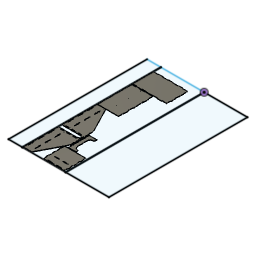
remorque marelle v9.1 v3 (Autodesk Fusion 360 design; units mm, degrees)
Autodesk Fusion 360 part; units mm, degrees
(part 1 of 2)
sketch "Esquisse1" plane through (0, 0, 0) normal (1, 0, 0) x (0, 0, -1)
  line L0 (0, 0) -> (0, 988)
  line L1 (0, 988) -> (-12, 988)
  line L2 (-12, 988) -> (-12, 0)
  line L3 (-12, 0) -> (0, 0)
  line L4 (605, 0) -> (0, 0)
  line L5 (180, 988) -> (192, 988)
  line L6 (192, 988) -> (192, 0)
  line L7 (192, 0) -> (180, 0)
  line L8 (180, 0) -> (180, 988)
  line L9 (-12, 988) -> (192, 988)
  line L10 (-12, 0) -> (605, 0)
  line L11 (605, 0) -> (605, -12)
  line L12 (605, -12) -> (-12, -12)
  line L13 (-12, -12) -> (-12, 0)
  line L14 (192, 988) -> (209.8465, 988)
  line L15 (227.5983, 977.2127) -> (569.8721, 317.6877)
  line L16 (605, 173.7399) -> (605, 0)
  arc A0 (227.5983, 977.2127) -> (209.8465, 988) centre (209.8465, 968) ccw
  arc A1 (605, 173.7399) -> (569.8721, 317.6877) centre (292.5, 173.7399) ccw
  line L17 (0, 988) -> (-12, 988)
  line L18 (-12, 988) -> (-12, 845.1428)
  line L19 (-12, 845.1428) -> (0, 845.1428)
  line L20 (0, 845.1428) -> (0, 988)
  line L21 (-12, 988) -> (-32.1287, 988)
  line L22 (-32.1287, 988) -> (-32.1287, -12)
  line L23 (-32.1287, -12) -> (-12, -12)
  line L24 (-12, -12) -> (-12, 988)
  line L25 (605, -12) -> (-32, -12)
  line L26 (-32, -12) -> (-32, -32)
  line L27 (-32, -32) -> (605, -32)
  line L28 (605, -32) -> (605, -12)
  line L29 (-32, -32) -> (-12, -32)
  line L30 (-12, -32) -> (-12, -12)
  line L31 (-12, -12) -> (-32, -12)
  line L32 (-32, -12) -> (-32, -32)
  line L33 (605, -32) -> (585, -32)
  line L34 (585, -32) -> (585, -12)
  line L35 (585, -12) -> (605, -12)
  line L36 (605, -12) -> (605, -32)
  line L37 (296.5, -12) -> (276.5, -12)
  line L38 (276.5, -12) -> (276.5, -32)
  line L39 (276.5, -32) -> (296.5, -32)
  line L40 (296.5, -32) -> (296.5, -12)
  line L41 (-12, 702.2857) -> (0, 702.2857)
  line L42 (0, 702.2857) -> (0, 845.1428)
  line L43 (-12, 845.1428) -> (-12, 702.2857)
  line L44 (0, 845.1428) -> (-12, 845.1428)
  line L45 (-12, 559.4286) -> (0, 559.4286)
  line L46 (0, 559.4286) -> (0, 702.2857)
  line L47 (-12, 702.2857) -> (-12, 559.4286)
  line L48 (0, 702.2857) -> (-12, 702.2857)
  line L49 (-12, 416.5714) -> (0, 416.5714)
  line L50 (0, 416.5714) -> (0, 559.4286)
  line L51 (-12, 559.4286) -> (-12, 416.5714)
  line L52 (0, 559.4286) -> (-12, 559.4286)
  line L53 (-12, 273.7143) -> (0, 273.7143)
  line L54 (0, 273.7143) -> (0, 416.5714)
  line L55 (-12, 416.5714) -> (-12, 273.7143)
  line L56 (0, 416.5714) -> (-12, 416.5714)
  line L57 (-12, 130.8571) -> (0, 130.8571)
  line L58 (0, 130.8571) -> (0, 273.7143)
  line L59 (-12, 273.7143) -> (-12, 130.8571)
  line L60 (0, 273.7143) -> (-12, 273.7143)
  line L61 (90, 988) -> (90, 0) construction
  line L62 (192, 130.8571) -> (180, 130.8571)
  line L63 (180, 273.7143) -> (192, 273.7143)
  line L64 (180, 416.5714) -> (192, 416.5714)
  line L65 (192, 559.4286) -> (180, 559.4286)
  line L66 (180, 702.2857) -> (192, 702.2857)
  line L67 (180, 845.1428) -> (192, 845.1428)
  line L68 (192, 0) -> (180, 0)
  line L69 (180, 0) -> (180, -12)
  line L70 (180, -12) -> (192, -12)
  line L71 (192, -12) -> (192, 0)
  line L72 (0, 0) -> (0, -12)
  line L73 (605, 0) -> (514, 0)
  line L74 (514, 0) -> (514, -12)
  line L75 (514, -12) -> (605, -12)
  line L76 (605, -12) -> (605, 0)
  line L77 (423, 0) -> (423, -12)
  line L78 (514, -12) -> (514, 0)
  line L79 (332, 0) -> (332, -12)
  line L80 (423, -12) -> (423, 0)
  line L81 (241, 0) -> (241, -12)
  line L82 (332, -12) -> (332, 0)
  line L83 (150, 0) -> (150, -12)
  line L84 (241, -12) -> (241, 0)
  line L85 (59, 0) -> (59, -12)
  line L86 (150, -12) -> (150, 0)
  line L87 (-32, 0) -> (-32, -12)
  line L88 (59, -12) -> (59, 0)
  line L89 (605, 173.7399) -> (593, 173.7399)
  line L90 (593, 173.7399) -> (593, -12)
  line L91 (593, -12) -> (605, -12)
  line L92 (605, -12) -> (605, 173.7399)
  line L93 (593, 173.7399) -> (605, 173.7399)
  line L94 (605, 173.7399) -> (605, 158.7399)
  line L95 (605, 158.7399) -> (593, 158.7399)
  line L96 (593, 158.7399) -> (593, 173.7399)
  line L97 (-12, 0) -> (-32, 0)
  circle A2 centre (-6, 973) radius 2
  circle A3 centre (-6, 860.1428) radius 2
  circle A4 centre (-6, 717.2857) radius 2
  circle A5 centre (-6, 830.1428) radius 2
  circle A6 centre (-6, 574.4286) radius 2
  circle A7 centre (-6, 687.2857) radius 2
  circle A8 centre (-6, 431.5714) radius 2
  circle A9 centre (-6, 544.4286) radius 2
  circle A10 centre (-6, 288.7143) radius 2
  circle A11 centre (-6, 401.5714) radius 2
  circle A12 centre (-6, 145.8571) radius 2
  circle A13 centre (-6, 258.7143) radius 2
  line L98 (-12, -12) -> (0, -12)
  line L99 (0, -12) -> (0, 130.8571)
  line L100 (-12, 130.8571) -> (-12, -12)
  line L101 (0, 130.8571) -> (-12, 130.8571)
  circle A14 centre (-6, 115.8571) radius 2
  circle A15 centre (186, 973) radius 2
  circle A16 centre (186, 860.1428) radius 2
  circle A17 centre (186, 687.2857) radius 2
  circle A18 centre (186, 574.4286) radius 2
  circle A19 centre (186, 401.5714) radius 2
  circle A20 centre (186, 288.7143) radius 2
  circle A21 centre (186, 115.8571) radius 2
  circle A22 centre (186, 15) radius 2
  circle A23 centre (-6, 15) radius 2
  line L102 (605, -6) -> (-32, -6) construction
  circle A24 centre (-20.1287, -6) radius 2
  circle A25 centre (47, -6) radius 2
  circle A26 centre (70.8713, -6) radius 2
  circle A27 centre (138, -6) radius 2
  circle A28 centre (161.8713, -6) radius 2
  circle A29 centre (229, -6) radius 2
  circle A30 centre (252.8713, -6) radius 2
  circle A31 centre (320, -6) radius 2
  circle A32 centre (343.8713, -6) radius 2
  circle A33 centre (411, -6) radius 2
  circle A34 centre (434.8713, -6) radius 2
  circle A35 centre (502, -6) radius 2
  circle A36 centre (525.8713, -6) radius 2
  circle A37 centre (593, -6) radius 2
  circle A38 centre (581, -6) radius 2
  line L103 (599, 158.7399) -> (593, 158.7399)
  line L104 (593, 158.7399) -> (593, 150.7399)
  line L105 (593, 150.7399) -> (599, 150.7399)
  line L106 (599, 150.7399) -> (599, 158.7399)
  point P0 (222, 988)
  point P1 (605, 250)
  dimension "d1" = 12
  dimension "d5" = 12
  dimension "d6" = 180
  dimension "d7" = 413
  dimension "d8" = 12
  dimension "d9" = 250
  dimension "d10" = 30
  dimension "d11" = 20
  dimension "d12" = 312.5
  dimension "d15" = 142.8571
  dimension "d17" = 20
  dimension "d18" = 20
  dimension "d19" = 20
  dimension "d22" = 0
  dimension "d23" = -142.8571
  dimension "d24" = 20
  dimension "d25" = 1020
  dimension "d28" = 91
  dimension "d31" = -91
  dimension "d32" = 0
  dimension "d44" = 12
  dimension "d47" = 15
  dimension "d56" = 4
  dimension "d57" = 6
  dimension "d58" = 15
  dimension "d59" = 4
  dimension "d60" = 15
  dimension "d61" = 6
  dimension "d62" = 4
  dimension "d63" = 15
  dimension "d64" = 4
  dimension "d65" = 15
  dimension "d66" = 4
  dimension "d67" = 4
  dimension "d68" = 12
  dimension "d69" = 12
  dimension "d72" = 91
  dimension "d73" = 0
  dimension "d74" = 4
  dimension "d75" = 12
  dimension "d103" = 8
  constraint coincident L0.start L3.end
  constraint vertical L0
  constraint perpendicular L0 L1
  constraint perpendicular L1 L2
  constraint perpendicular L0 L3
  constraint perpendicular L0 L4
  constraint horizontal L5
  constraint vertical L6
  constraint horizontal L7
  constraint vertical L8
  constraint coincident L4 L6.end
  constraint perpendicular L6 L9
  constraint horizontal L10
  constraint vertical L11
  constraint horizontal L12
  constraint vertical L13
  constraint perpendicular L6 L14
  constraint perpendicular L10 L16
  constraint coincident P0 L14
  constraint coincident P0 L15
  constraint tangent L14 A0
  constraint tangent L15 A0
  constraint coincident P1 L15
  constraint coincident P1 L16
  constraint tangent L15 A1
  constraint tangent L16 A1
  constraint horizontal L17
  constraint vertical L18
  constraint horizontal L19
  constraint vertical L20
  constraint coincident L2 L18.end
  constraint horizontal L21
  constraint vertical L22
  constraint horizontal L23
  constraint vertical L24
  constraint horizontal L25
  constraint vertical L26
  constraint horizontal L27
  constraint vertical L28
  constraint horizontal L29
  constraint vertical L30
  constraint horizontal L31
  constraint vertical L32
  constraint horizontal L33
  constraint vertical L34
  constraint horizontal L35
  constraint vertical L36
  constraint horizontal L37
  constraint vertical L38
  constraint horizontal L39
  constraint vertical L40
  constraint coincident L12 L37.start
  constraint midpoint L27 L39
  constraint midpoint L9 L61.start
  constraint coincident L10 L61.end
  constraint perpendicular L4 L61
  constraint symmetric L19.end L61 L67.start
  constraint symmetric L18.end L61 L67.end
  constraint symmetric L45.start L61 L65.start
  constraint symmetric L45.end L61 L65.end
  constraint symmetric L41.end L61 L66.start
  constraint symmetric L41.start L61 L66.end
  constraint symmetric L49.end L61 L64.start
  constraint symmetric L49.start L61 L64.end
  constraint symmetric L57.start L61 L62.start
  constraint symmetric L57.end L61 L62.end
  constraint symmetric L53.end L61 L63.start
  constraint symmetric L53.start L61 L63.end
  constraint horizontal L68
  constraint vertical L69
  constraint horizontal L70
  constraint vertical L71
  constraint coincident L25 L69.end
  constraint coincident L7.end L8.start
  constraint coincident L12 L72.end
  constraint collinear L0 L72
  constraint horizontal L73
  constraint vertical L74
  constraint horizontal L75
  constraint vertical L76
  constraint coincident L25 L74.end
  constraint coincident L4.start L10.end
  constraint horizontal L89
  constraint vertical L90
  constraint horizontal L91
  constraint vertical L92
  constraint coincident L25 L90.end
  constraint coincident L35 L90.end
  constraint horizontal L93
  constraint vertical L94
  constraint horizontal L95
  constraint vertical L96
  constraint symmetric L61 A2 A15
  constraint symmetric L61 A3 A16
  constraint symmetric L61 A6 A18
  constraint symmetric L61 A7 A17
  constraint symmetric L61 A10 A20
  constraint symmetric L61 A11 A19
  constraint symmetric L61 A14 A21
  constraint midpoint L11 L102.start
  constraint midpoint L87 L102.end
  constraint coincident L102 A24.centre
  constraint coincident L102 A25.centre
  constraint coincident L102 A38.centre
  constraint horizontal L103
  constraint vertical L104
  constraint horizontal L105
  constraint vertical L106
  constraint coincident L90 L104.end
  constraint midpoint L95 L103.start
  measures "d1" distance of L2.end L0.start
  measures "d5" distance of L6 L8
  measures "d6" distance of L0 L8
  measures "d7" distance of L4.start L6
  measures "d8" distance of L10 L12
  measures "d9" distance of L4.start P1
  measures "d10" distance of L5.end P0
  measures "d11" radius of A0
  measures "d12" radius of A1
  measures "d15" distance of L0.end L19.end
  measures "d17" distance of L25 L27
  measures "d18" distance of L27.end L33.end
  measures "d19" distance of L38 L40
  measures "d24" distance of L26 L30
  measures "d25" distance of L21.end L26.end
  measures "d28" distance of L74 L76
  measures "d44" distance of L16 L90
  measures "d47" distance of L89.end L95.end
  measures "d56" diameter of A2
  measures "d57" distance of L18 A2.centre
  measures "d58" distance of L9 A2.centre
  measures "d59" diameter of A3
  measures "d60" distance of L44 A3.centre
  measures "d61" distance of L18 A3.centre
  measures "d62" diameter of A22
  measures "d63" distance of L68 A22.centre
  measures "d64" diameter of A23
  measures "d65" distance of L3 A23.centre
  measures "d66" diameter of A24
  measures "d67" diameter of A25
  measures "d68" distance of L85 A25.centre
  measures "d69" distance of L22 A24.centre
  measures "d74" diameter of A38
  measures "d75" distance of A37.centre A38.centre
  measures "d103" distance of L103.start L105.end
sketch "Esquisse2" plane through (0, 0, 0) normal (1, 0, 0) x (0, 0, -1)
  line L0 (605, -12) -> (-32, -12)
  line L1 (-32, -32) -> (605, -32)
  line L2 (-12, 0) -> (605, 0)
  line L3 (-32, 0) -> (-32, -12)
  line L4 (-32, -12) -> (-32, -32)
  line L5 (605, -12) -> (605, -32)
  line L6 (605, 0) -> (605, -12)
  line L7 (-12, -32) -> (113, -32)
  line L8 (113, -32) -> (113, -42)
  line L9 (113, -42) -> (-12, -42)
  line L10 (-12, -42) -> (-12, -32)
  circle A0 centre (50.5, -57) radius 15
  circle A1 centre (50.5, -57) radius 4
  circle A2 centre (50.5, -57) radius 200
  line L11 (50.5, -57) -> (50.5, -42)
  line L12 (50.5, -257) -> (650, -257)
  line L13 (593, -12) -> (605, 0)
  line L14 (593, 173.7399) -> (593, -12)
  line L15 (593, 0) -> (605, -12)
  line L16 (605, -12) -> (605, 173.7399)
  line L17 (605, 173.7399) -> (593, 173.7399)
  line L18 (593, 0) -> (605, 0)
  line L19 (605, 0) -> (605, -257)
  line L20 (605, -257) -> (593, -257)
  line L21 (593, -257) -> (593, 0)
  line L22 (599, 173.7399) -> (599, -257)
  line L23 (605, -48.13) -> (593, -48.13)
  line L24 (593, -48.13) -> (593, -35.13)
  line L25 (593, -35.13) -> (605, -35.13)
  line L26 (605, -35.13) -> (605, -48.13)
  circle A3 centre (599, -41.63) radius 8.8459
  circle A4 centre (599, -41.63) radius 30
  line L27 (626.1765, -28.9242) -> (605, 16.37)
  line L28 (585.3674, -68.3537) -> (514.1044, -32)
  line L29 (593, -48.13) -> (605, -48.13)
  line L30 (605, -48.13) -> (605, -56.13)
  line L31 (605, -56.13) -> (593, -56.13)
  line L32 (593, -56.13) -> (593, -48.13)
  line L33 (593, -35.13) -> (605, -35.13)
  line L34 (605, -35.13) -> (605, -27.13)
  line L35 (605, -27.13) -> (593, -27.13)
  line L36 (593, -27.13) -> (593, -35.13)
  line L37 (593, -27.13) -> (605, -27.13)
  line L38 (605, -27.13) -> (605, -35.13)
  line L39 (605, -35.13) -> (593, -35.13)
  line L40 (593, -35.13) -> (593, -27.13)
  line L41 (593, -48.13) -> (605, -48.13)
  line L42 (605, -48.13) -> (605, -56.13)
  line L43 (605, -56.13) -> (593, -56.13)
  line L44 (593, -56.13) -> (593, -48.13)
  line L45 (605, -35.63) -> (593, -35.63)
  line L46 (593, -35.63) -> (593, -47.63)
  line L47 (593, -47.63) -> (605, -47.63)
  line L48 (605, -47.63) -> (605, -35.63)
  line L49 (605, -35.63) -> (593, -47.63) construction
  point P0 (-32, -32)
  point P1 (50.5, -42)
  point P2 (593, -12)
  point P3 (599, -6)
  point P4 (599, -41.63)
  point P5 (599, -41.63)
  dimension "d38" = 20
  dimension "d39" = 10
  dimension "d40" = 30
  dimension "d41" = 8
  dimension "d42" = 400
  dimension "d43" = 125
  dimension "d45" = 13
  dimension "d46" = 60
  dimension "d48" = 50
  dimension "d49" = 80
  dimension "d99" = 8
  dimension "d100" = 8
  dimension "d110" = 12
  dimension "d111" = 12
  constraint horizontal L7
  constraint vertical L8
  constraint horizontal L9
  constraint vertical L10
  constraint coincident L1 L7.start
  constraint tangent L9 A0
  constraint concentric A0 A1
  constraint concentric A0 A2
  constraint coincident A0.centre A1.centre
  constraint coincident A0 P1
  constraint perpendicular L9 L11
  constraint midpoint L9 P1
  constraint coincident P1 L11.end
  constraint coincident A2 L12.start
  constraint horizontal L12
  constraint tangent A2 L12
  constraint coincident L0 P2
  constraint coincident L2.end L6.start
  constraint coincident P2 L13.start
  constraint coincident L14 L15.start
  constraint coincident L2 L15.start
  constraint coincident L0.start L5.start
  constraint midpoint L15 P3
  constraint horizontal L18
  constraint vertical L19
  constraint horizontal L20
  constraint vertical L21
  constraint coincident L12 L19.end
  constraint midpoint L17 L22.start
  constraint midpoint L20 L22.end
  constraint perpendicular L20 L22
  constraint midpoint L22 P5
  constraint horizontal L23
  constraint perpendicular L23 L24
  constraint parallel L23 L25
  constraint parallel L24 L26
  constraint coincident P5 P4
  constraint coincident L25.end A3
  constraint coincident A4 L27.start
  constraint coincident L16 L27.end
  constraint tangent A4 L27
  constraint coincident A4 L28.start
  constraint coincident L1 L28.end
  constraint tangent A4 L28
  constraint horizontal L29
  constraint vertical L30
  constraint horizontal L31
  constraint vertical L32
  constraint coincident L19 L30.end
  constraint horizontal L33
  constraint vertical L34
  constraint horizontal L35
  constraint vertical L36
  constraint coincident L5 L34.end
  constraint horizontal L37
  constraint vertical L38
  constraint horizontal L39
  constraint vertical L40
  constraint horizontal L41
  constraint vertical L42
  constraint horizontal L43
  constraint vertical L44
  constraint coincident L21 L35.end
  constraint horizontal L45
  constraint vertical L46
  constraint horizontal L47
  constraint vertical L48
  constraint midpoint P5 L49
  measures "d38" distance of L7.start P0
  measures "d39" distance of L7.end L8.end
  measures "d40" diameter of A0
  measures "d41" diameter of A1
  measures "d42" diameter of A2
  measures "d43" distance of L8.end L9.end
  measures "d45" distance of L23.end L24.end
  measures "d46" diameter of A4
  measures "d48" distance of L27.start L27.end
  measures "d49" distance of L28.start L28.end
  measures "d99" distance of L25 L35
  measures "d100" distance of L29 L31
  measures "d110" distance of L46.end L47.end
  measures "d111" distance of L45.end L46.end
extrude "Extrusion2" add sketch "Esquisse2" sketch "Esquisse1" along normal blind 12 contours L5 L6 L16 L19 A4 L27 | L5 L19 A3 A4 L30 L34 L38 L42 | L1 L19 L22 A3 L34 L38 | L1 L21 L22 A3 L36 L40 | L19 L22 A4 L31 L43 | L1 A4 L28 | L1 L21 A3 A4 L32 L36 L40 L44 | L19 L22 A3 L30 L31 L42 L43 | L21 L22 A4 L31 L43 | L21 L22 A3 L31 L32 L43 L44 of sketch 2 contours L0 L2 L3 L10 L24 L57 L99 L100 L101 | L3 L10 L12 L13 L24 L25 L72 L98 L99 L100 | L0 L4 L8 L9 L10 L20 L42 L46 L50 L54 L58 L99 | L4 L10 L12 L25 L72 L85 L88 L99 | L0 L2 L24 L53 L57 L58 L59 L60 L101 | L2 L18 L21 L22 L23 L24 L43 L47 L51 L55 L59 L87 L97 L100 | L13 L23 L24 L25 L31 L87 L97 L100 | L4 L10 L12 L25 L83 L85 L86 L88 | L12 L25 L27 L30 L38 L70 L98 | L0 L2 L24 L49 L53 L54 L55 L56 L60 | L23 L25 L26 L27 L29 L30 L31 L32 | L4 L10 L12 L25 L69 L83 L86 | L0 L2 L24 L45 L49 L50 L51 L52 L56 | L4 L6 L7 L8 L10 L62 L68 | L4 L7 L10 L12 L25 L68 L69 L70 L71 | L0 L2 L24 L41 L45 L46 L47 L48 L52 | L12 L25 L27 L37 L38 L39 L40 | L4 L6 L10 L14 L15 A0 A1 L73 L89 L90 L93 L96 L104 | L4 L10 L12 L25 L71 L81 L84 | L6 L8 L62 L63 | L0 L2 L19 L24 L41 L42 L43 L44 L48 | L12 L25 L27 L34 L40 L75 | L4 L10 L12 L25 L37 L79 L81 L82 L84 | L6 L8 L63 L64 | L0 L1 L2 L9 L17 L18 L19 L20 L24 L44 | L12 L25 L27 L28 L33 L34 L35 L36 L75 L91 | L4 L10 L12 L25 L77 L79 L80 L82 | L6 L8 L64 L65 | L4 L10 L12 L25 L35 L73 L74 L75 L78 L90 A37 | L4 L10 L12 L25 L74 L77 L78 L80 | L6 L8 L65 L66 | L5 L6 L8 L9 L67 | L4 L10 L11 L12 L25 L35 L73 L75 L76 L90 L91 L92 A37 | L6 L8 L66 L67 | L4 L10 L16 L73 L90 L92 L95 L105 L106 | L90 A37 | L90 A37 | A4 | A5 | A8 | A9 | A12 | A13 | A26 | A27 | A30 | A31 | A34 | A35 makes body 1
extrude "Extrusion12" cut sketch "Esquisse2" along normal blind 12 contours L1 L5 L19 L22 L34 L35 L37 L38 | L1 L21 L22 L35 L36 L37 L40 | L1 L19 L22 A3 L34 L38 | L1 L21 L22 A3 L36 L40 | L19 L22 A3 L30 L31 L42 L43 | L22 L23 A3 L29 L41 | L21 L22 A3 L31 L32 L43 L44 | L22 L23 A3 L29 L41 bodies 1
sketch "Esquisse5" plane through (12, 0, 0) normal (1, 0, 0) x (0, 0, -1)
  arc A0 (585.3674, -68.3537) -> (626.1765, -28.9242) centre (599, -41.63) ccw
  line L0 (626.1765, -28.9242) -> (605, 16.37)
  line L1 (605, 16.37) -> (605, 158.7399)
  line L2 (605, 158.7399) -> (599, 158.7399)
  line L3 (599, 158.7399) -> (599, 150.7399)
  line L4 (599, 150.7399) -> (593, 150.7399)
  line L5 (593, 150.7399) -> (593, 158.7399)
  line L6 (593, 158.7399) -> (593, 173.7399)
  line L7 (593, 173.7399) -> (605, 173.7399)
  arc A1 (605, 173.7399) -> (569.8721, 317.6877) centre (292.5, 173.7399) ccw
  line L8 (569.8721, 317.6877) -> (227.5983, 977.2127)
  arc A2 (227.5983, 977.2127) -> (209.8465, 988) centre (209.8465, 968) ccw
  line L9 (209.8465, 988) -> (-32.1287, 988)
  line L10 (-32.1287, 988) -> (-32.1287, -12)
  line L11 (-32.1287, -12) -> (-32, -12)
  line L12 (-32, -12) -> (-32, -32)
  line L13 (-32, -32) -> (514.1044, -32)
  line L14 (514.1044, -32) -> (585.3674, -68.3537)
  circle A3 centre (47, -6) radius 2
  circle A4 centre (-20.1287, -6) radius 2
  circle A5 centre (186, 115.8571) radius 2
  circle A6 centre (186, 15) radius 2
  circle A7 centre (186, 574.4286) radius 2
  circle A8 centre (186, 401.5714) radius 2
  circle A9 centre (186, 973) radius 2
  circle A10 centre (186, 860.1428) radius 2
  circle A11 centre (186, 288.7143) radius 2
  circle A12 centre (-6, 973) radius 2
  circle A13 centre (-6, 15) radius 2
  circle A14 centre (411, -6) radius 2
  circle A15 centre (186, 687.2857) radius 2
  circle A16 centre (581, -6) radius 2
  circle A17 centre (525.8713, -6) radius 2
  circle A18 centre (-6, 860.1428) radius 2
  circle A19 centre (-6, 687.2857) radius 2
  circle A20 centre (-6, 574.4286) radius 2
  circle A21 centre (343.8713, -6) radius 2
  circle A22 centre (229, -6) radius 2
  circle A23 centre (-6, 401.5714) radius 2
  circle A24 centre (-6, 288.7143) radius 2
  circle A25 centre (161.8713, -6) radius 2
  circle A26 centre (-6, 115.8571) radius 2
  line L15 (605, -56.13) -> (593, -56.13)
  line L16 (593, -56.13) -> (593, -48.13)
  arc A27 (593, -35.13) -> (593, -48.13) centre (599, -41.63) ccw
  line L17 (593, -35.13) -> (593, -27.13)
  line L18 (593, -27.13) -> (605, -27.13)
  line L19 (605, -27.13) -> (605, -35.13)
  arc A28 (605, -48.13) -> (605, -35.13) centre (599, -41.63) ccw
  line L20 (605, 173.7399) -> (605, 158.7399)
  line L21 (605, -48.13) -> (605, -56.13)
  constraint coincident L7.end A1.start
  constraint coincident L1.end L2.start
extrude "Extrusion13" add sketch "Esquisse5" against normal blind 6 contours L2 L3 L4 L5 L6 L7 L20 bodies 1
extrude "Extrusion3" cut sketch "Esquisse1" along normal blind 12 contours L0 L2 L24 L53 L57 L58 L59 L60 L101 | L4 L10 L12 L25 L83 L85 L86 L88 | L0 L2 L24 L45 L49 L50 L51 L52 L56 | L6 L8 L62 L63 | L0 L2 L19 L24 L41 L42 L43 L44 L48 | L4 L10 L12 L25 L37 L79 L81 L82 L84 | L6 L8 L64 L65 | L4 L10 L12 L25 L74 L77 L78 L80 | L6 L8 L66 L67 | A4 | A5 | A8 | A9 | A12 | A13 | A26 | A27 | A30 | A31 | A34 | A35 bodies 1
ref_plane "Plan de construction1" through (-301, 494, -398.5) normal (1, 0, 0) x (0, 0, -1)
mirror "Symétrie miroir1" about plane through (-301, 494, -398.5) normal (1, 0, 0) of bodies 1 makes body 2
extrude "Extrusion4" add sketch "Esquisse1" against normal blind 602 separate body contours L3 L10 L12 L13 L24 L25 L72 L98 L99 L100 | L4 L10 L12 L25 L72 L85 L88 L99 | L13 L23 L24 L25 L31 L87 L97 L100 | L4 L10 L12 L25 L83 L85 L86 L88 | L4 L10 L12 L25 L69 L83 L86 | L4 L7 L10 L12 L25 L68 L69 L70 L71 | L4 L10 L12 L25 L71 L81 L84 | L4 L10 L12 L25 L37 L79 L81 L82 L84 | L4 L10 L12 L25 L77 L79 L80 L82 | L4 L10 L12 L25 L35 L73 L74 L75 L78 L90 A37 | L4 L10 L12 L25 L74 L77 L78 L80 | L90 A37 | A24 | A25 | A26 | A27 | A28 | A29 | A30 | A31 | A32 | A33 | A34 | A35 | A36 | A38 picked at (592.7107, -6.6006) makes body 3
extrude "Extrusion5" add sketch "Esquisse1" along normal blind 12 contours L4 L10 L12 L25 L83 L85 L86 L88 | L4 L10 L12 L25 L37 L79 L81 L82 L84 | L4 L10 L12 L25 L74 L77 L78 L80 | A26 | A27 | A30 | A31 | A34 | A35 bodies 3
sketch "Esquisse3" plane through (-602, 0, 0) normal (1, 0, 0) x (0, 0, -1)
  line L0 (59, -12) -> (59, 0)
  line L1 (59, 0) -> (150, 0)
  line L2 (150, 0) -> (150, -12)
  line L3 (150, -12) -> (59, -12)
  line L4 (180, 273.7143) -> (192, 273.7143)
  line L5 (192, 273.7143) -> (192, 130.8571)
  line L6 (192, 130.8571) -> (180, 130.8571)
  line L7 (180, 130.8571) -> (180, 273.7143)
  line L8 (180, 416.5714) -> (180, 559.4286)
  line L9 (180, 559.4286) -> (192, 559.4286)
  line L10 (192, 559.4286) -> (192, 416.5714)
  line L11 (192, 416.5714) -> (180, 416.5714)
  line L12 (0, 845.1428) -> (0, 702.2857)
  line L13 (0, 702.2857) -> (-12, 702.2857)
  line L14 (-12, 702.2857) -> (-12, 845.1428)
  line L15 (-12, 845.1428) -> (0, 845.1428)
  line L16 (241, -12) -> (241, 0)
  line L17 (241, 0) -> (332, 0)
  line L18 (332, 0) -> (332, -12)
  line L19 (332, -12) -> (241, -12)
  line L20 (0, 273.7143) -> (0, 130.8571)
  line L21 (0, 130.8571) -> (-12, 130.8571)
  line L22 (-12, 130.8571) -> (-12, 273.7143)
  line L23 (-12, 273.7143) -> (0, 273.7143)
  line L24 (180, 702.2857) -> (180, 845.1428)
  line L25 (180, 845.1428) -> (192, 845.1428)
  line L26 (192, 845.1428) -> (192, 702.2857)
  line L27 (192, 702.2857) -> (180, 702.2857)
  line L28 (0, 559.4286) -> (0, 416.5714)
  line L29 (0, 416.5714) -> (-12, 416.5714)
  line L30 (-12, 416.5714) -> (-12, 559.4286)
  line L31 (-12, 559.4286) -> (0, 559.4286)
  line L32 (423, -12) -> (423, 0)
  line L33 (423, 0) -> (514, 0)
  line L34 (514, 0) -> (514, -12)
  line L35 (514, -12) -> (423, -12)
  arc A0 (585.3674, -68.3537) -> (626.1765, -28.9242) centre (599, -41.63) ccw
  line L36 (626.1765, -28.9242) -> (605, 16.37)
  line L37 (605, 16.37) -> (605, 158.7399)
  line L38 (605, 158.7399) -> (599, 158.7399)
  line L39 (593, 173.7399) -> (605, 173.7399)
  arc A1 (605, 173.7399) -> (569.8721, 317.6877) centre (292.5, 173.7399) ccw
  line L40 (569.8721, 317.6877) -> (227.5983, 977.2127)
  arc A2 (227.5983, 977.2127) -> (209.8465, 988) centre (209.8465, 968) ccw
  line L41 (209.8465, 988) -> (-32.1287, 988)
  line L42 (-32.1287, 988) -> (-32.1287, -12)
  line L43 (-32.1287, -12) -> (-32, -12)
  line L44 (-32, -12) -> (-32, -32)
  line L45 (-32, -32) -> (514.1044, -32)
  line L46 (514.1044, -32) -> (585.3674, -68.3537)
  circle A3 centre (186, 288.7143) radius 2
  circle A4 centre (-6, 401.5714) radius 2
  circle A5 centre (-6, 973) radius 2
  circle A6 centre (-6, 687.2857) radius 2
  circle A7 centre (-6, 574.4286) radius 2
  circle A8 centre (-6, 288.7143) radius 2
  circle A9 centre (-6, 860.1428) radius 2
  circle A10 centre (-6, 115.8571) radius 2
  circle A11 centre (186, 860.1428) radius 2
  circle A12 centre (186, 401.5714) radius 2
  circle A13 centre (186, 687.2857) radius 2
  circle A14 centre (186, 574.4286) radius 2
  circle A15 centre (186, 973) radius 2
  circle A16 centre (186, 115.8571) radius 2
  circle A17 centre (186, 15) radius 2
  circle A18 centre (-6, 15) radius 2
  circle A19 centre (581, -6) radius 2
  circle A20 centre (47, -6) radius 2
  circle A21 centre (161.8713, -6) radius 2
  circle A22 centre (525.8713, -6) radius 2
  circle A23 centre (411, -6) radius 2
  circle A24 centre (343.8713, -6) radius 2
  circle A25 centre (229, -6) radius 2
  circle A26 centre (-20.1287, -6) radius 2
  line L47 (593, -35.13) -> (593, -27.13)
  line L48 (593, -27.13) -> (605, -27.13)
  line L49 (605, -27.13) -> (605, -35.13)
  arc A27 (605, -48.13) -> (605, -35.13) centre (599, -41.63) ccw
  line L50 (605, -56.13) -> (593, -56.13)
  line L51 (593, -56.13) -> (593, -48.13)
  arc A28 (593, -35.13) -> (593, -48.13) centre (599, -41.63) ccw
  line L52 (599, 158.7399) -> (599, 150.7399)
  line L53 (599, 150.7399) -> (593, 150.7399)
  line L54 (593, 150.7399) -> (593, 158.7399)
  line L55 (605, -48.13) -> (605, -56.13)
  line L56 (593, 158.7399) -> (593, 173.7399)
extrude "Extrusion6" add sketch "Esquisse3" against normal blind 12 contours L0 L1 L2 L3 | L16 L17 L18 L19 | L32 L33 L34 L35 bodies 3
extrude "Extrusion7" add sketch "Esquisse1" against normal blind 602 separate body contours L0 L2 L3 L10 L24 L57 L99 L100 L101 | L0 L2 L24 L53 L57 L58 L59 L60 L101 | L0 L2 L24 L49 L53 L54 L55 L56 L60 | L0 L2 L24 L45 L49 L50 L51 L52 L56 | L4 L6 L7 L8 L10 L62 L68 | L0 L2 L24 L41 L45 L46 L47 L48 L52 | L6 L8 L62 L63 | L0 L2 L19 L24 L41 L42 L43 L44 L48 | L6 L8 L63 L64 | L0 L1 L2 L9 L17 L18 L19 L20 L24 L44 | L6 L8 L64 L65 | L6 L8 L65 L66 | L5 L6 L8 L9 L67 | L6 L8 L66 L67 | A2 | A3 | A4 | A5 | A6 | A7 | A8 | A9 | A10 | A11 | A12 | A13 | A14 | A15 | A16 | A17 | A18 | A19 | A20 | A21 | A22 | A23 makes body 4 at (-401.3333, 329.3333, -180) makes body 5 at (-200.6667, 658.6667, 12)
extrude "Extrusion8" add sketch "Esquisse1" along normal blind 12 contours L0 L2 L24 L53 L57 L58 L59 L60 L101 | L0 L2 L24 L45 L49 L50 L51 L52 L56 | L6 L8 L62 L63 | L0 L2 L19 L24 L41 L42 L43 L44 L48 | L6 L8 L64 L65 | L6 L8 L66 L67 | A4 | A5 | A8 | A9 | A12 | A13 bodies 4 5
extrude "Extrusion9" add sketch "Esquisse3" against normal blind 12 contours L4 L5 L6 L7 | L8 L9 L10 L11 | L12 L13 L14 L15 | L20 L21 L22 L23 | L24 L25 L26 L27 | L28 L29 L30 L31 bodies 4 5
sketch "Esquisse4" plane through (0, 0, 0) normal (0, -1, 0) x (1, 0, 0)
  line L0 (0, 0) -> (0, 12)
  line L1 (0, 12) -> (-602, 12)
  line L2 (-602, 12) -> (-602, 0)
  line L3 (-602, 0) -> (0, 0)
  line L4 (0, -192) -> (0, -180)
  line L5 (0, -180) -> (-602, -180)
  line L6 (-602, -180) -> (-602, -192)
  line L7 (-602, -192) -> (0, -192)
  line L8 (-602, 0) -> (-614, 0)
  line L9 (-614, 0) -> (-614, 12)
  line L10 (-614, 12) -> (-602, 12)
  line L11 (-602, 12) -> (-602, 0)
  line L12 (0, 0) -> (12, 0)
  line L13 (12, 0) -> (12, 12)
  line L14 (12, 12) -> (0, 12)
  line L15 (0, 12) -> (0, 0)
  line L16 (0, -192) -> (12, -192)
  line L17 (12, -192) -> (12, -180)
  line L18 (12, -180) -> (0, -180)
  line L19 (0, -180) -> (0, -192)
  line L20 (-602, -192) -> (-614, -192)
  line L21 (-614, -192) -> (-614, -180)
  line L22 (-614, -180) -> (-602, -180)
  line L23 (-602, -180) -> (-602, -192)
  line L24 (-614, -514.1044) -> (-602, -514.1044)
  line L25 (-602, -514.1044) -> (-602, 32)
  line L26 (-602, 32) -> (-614, 32)
  line L27 (-614, 32) -> (-614, -514.1044)
  line L28 (0, -514.1044) -> (12, -514.1044)
  line L29 (12, -514.1044) -> (12, 32)
  line L30 (12, 32) -> (0, 32)
  line L31 (0, 32) -> (0, -514.1044)
  line L32 (-614, -180) -> (-488.8, -180)
  line L33 (-488.8, -180) -> (-488.8, -192)
  line L34 (-488.8, -192) -> (-614, -192)
  line L35 (-614, -192) -> (-614, -180)
  line L36 (-363.6, -180) -> (-363.6, -192)
  line L37 (-488.8, -180) -> (-363.6, -180)
  line L38 (-363.6, -192) -> (-488.8, -192)
  line L39 (-488.8, -192) -> (-488.8, -180)
  line L40 (-238.4, -180) -> (-238.4, -192)
  line L41 (-363.6, -180) -> (-238.4, -180)
  line L42 (-238.4, -192) -> (-363.6, -192)
  line L43 (-363.6, -192) -> (-363.6, -180)
  line L44 (-113.2, -180) -> (-113.2, -192)
  line L45 (-238.4, -180) -> (-113.2, -180)
  line L46 (-113.2, -192) -> (-238.4, -192)
  line L47 (-238.4, -192) -> (-238.4, -180)
  line L48 (12, -180) -> (12, -192)
  line L49 (-113.2, -180) -> (12, -180)
  line L50 (12, -192) -> (-113.2, -192)
  line L51 (-113.2, -192) -> (-113.2, -180)
  line L52 (-602, 0) -> (-602, -180)
  line L53 (-602, -90) -> (12, -90)
  line L54 (-488.8, 0) -> (-488.8, 12)
  line L55 (-363.6, 0) -> (-363.6, 12)
  line L56 (-238.4, 12) -> (-238.4, 0)
  line L57 (-113.2, 12) -> (-113.2, 0)
  circle A0 centre (-8, -186) radius 2
  circle A1 centre (-93.2, -186) radius 2
  circle A2 centre (-258.4, -186) radius 2
  circle A3 centre (-343.6, -186) radius 2
  circle A4 centre (-508.8, -186) radius 2
  circle A5 centre (-594, -186) radius 2
  circle A6 centre (-8, 6) radius 2
  circle A7 centre (-343.6, 6) radius 2
  circle A8 centre (-258.4, 6) radius 2
  circle A9 centre (-508.8, 6) radius 2
  circle A10 centre (-594, 6) radius 2
  circle A11 centre (-93.2, 6) radius 2
  circle A12 centre (-301, 24.6) radius 12.6
  line L58 (-602, 24.6) -> (0, 24.6)
  line L59 (-313.6, 24.6) -> (-313.6, 30)
  line L60 (-313.6, 30) -> (-313.6, 32)
  line L61 (0, -514) -> (0, -593)
  line L62 (0, -593) -> (-602, -593)
  line L63 (-602, -593) -> (-602, -514)
  line L64 (-602, -514) -> (-614, -514)
  line L65 (-614, -514) -> (-614, -423)
  line L66 (-614, -423) -> (-602, -423)
  line L67 (-602, -423) -> (-602, -332)
  line L68 (-602, -332) -> (-614, -332)
  line L69 (-614, -332) -> (-614, -241)
  line L70 (-614, -241) -> (-602, -241)
  line L71 (-602, -241) -> (-602, -150)
  line L72 (-602, -150) -> (-614, -150)
  line L73 (-614, -150) -> (-614, -59)
  line L74 (-614, -59) -> (-602, -59)
  line L75 (-602, -59) -> (-602, 32)
  line L76 (-602, 32) -> (0, 32)
  line L77 (0, 32) -> (0, -59)
  line L78 (0, -59) -> (12, -59)
  line L79 (12, -59) -> (12, -150)
  line L80 (12, -150) -> (0, -150)
  line L81 (0, -150) -> (0, -241)
  line L82 (0, -241) -> (12, -241)
  line L83 (12, -241) -> (12, -332)
  line L84 (12, -332) -> (0, -332)
  line L85 (0, -332) -> (0, -423)
  line L86 (0, -423) -> (12, -423)
  line L87 (12, -423) -> (12, -514)
  line L88 (12, -514) -> (0, -514)
  line L89 (-288.4, 24.6) -> (-288.4, 32)
  point P0 (-93.2, 6)
  dimension "d82" = 125.2
  dimension "d85" = 125.2
  dimension "d86" = 0
  dimension "d89" = 4
  dimension "d90" = 4
  dimension "d91" = 20
  dimension "d92" = 20
  dimension "d95" = -250.4
  dimension "d96" = 0
  dimension "d260" = 25.2
  constraint horizontal L8
  constraint vertical L9
  constraint horizontal L10
  constraint vertical L11
  constraint coincident L2.end L3.start
  constraint horizontal L12
  constraint vertical L13
  constraint horizontal L14
  constraint vertical L15
  constraint coincident L0.start L3.end
  constraint horizontal L16
  constraint vertical L17
  constraint horizontal L18
  constraint vertical L19
  constraint coincident L4.start L7.end
  constraint horizontal L20
  constraint vertical L21
  constraint horizontal L22
  constraint vertical L23
  constraint coincident L6.end L7.start
  constraint coincident L12.end L29
  constraint coincident L8.end L27
  constraint coincident L20.end L27
  constraint coincident L17.end L29
  constraint horizontal L32
  constraint vertical L33
  constraint horizontal L34
  constraint vertical L35
  constraint coincident L7 L33.end
  constraint coincident L5.end L6.start
  constraint midpoint L52 L53.start
  constraint coincident L29 L53.end
  constraint perpendicular L29 L53
  constraint symmetric L32.end L53 L54.start
  constraint symmetric L33.end L53 L54.end
  constraint symmetric L36.start L53 L55.start
  constraint symmetric L36.end L53 L55.end
  constraint symmetric L40.start L53 L56.end
  constraint symmetric L40.end L53 L56.start
  constraint symmetric L44.start L53 L57.end
  constraint symmetric L44.end L53 L57.start
  constraint symmetric L53 A0 A6
  constraint symmetric L53 A1.centre P0
  constraint symmetric L53 A2 A8
  constraint symmetric L53 A3 A7
  constraint symmetric L53 A4 A9
  constraint symmetric L53 A5 A10
  constraint symmetric L53 A1 A11
  constraint tangent L1 A12
  constraint coincident L25 L58.start
  constraint coincident L31 L58.end
  constraint perpendicular L31 L58
  constraint midpoint A12.centre L58
  constraint coincident A12 L59.start
  constraint coincident L58 L59.start
  constraint tangent A12 L59
  constraint perpendicular L1 L60
  constraint coincident L60.end L76
  constraint coincident A12 L89.start
  constraint coincident L58 L89.start
  constraint coincident L76 L89.end
  constraint tangent A12 L89
  measures "d82" distance of L33 L35
  measures "d89" diameter of A0
  measures "d90" diameter of A1
  measures "d91" distance of L48 A0.centre
  measures "d92" distance of L51 A1.centre
  measures "d260" diameter of A12
extrude "Extrusion10" add sketch "Esquisse4" along normal blind 12 contours L1 L3 L56 L57 | L1 L3 L54 L55 | L5 L7 L40 L44 L45 L46 L47 L51 | L5 L7 L33 L36 L37 L38 L39 L43 bodies 5 4
combine "Combiner1" operation cut target body 3 tool bodies 4 keep tools
combine "Combiner2" operation cut target body 3 tool bodies 5 keep tools
extrude "Extrusion11" cut sketch "Esquisse4" along normal blind 12 contours A0 | A1 | A2 | A3 | A4 | A5 | A6 | A7 | A8 | A9 | A10 | A11 bodies 3
sketch "Esquisse6" plane through (0, 0, -593) normal (0, 0, -1) x (-1, 0, 0)
  line L0 (-6, 173.7399) -> (-6, 158.7399)
  line L1 (-6, 158.7399) -> (0, 158.7399)
  line L2 (0, 158.7399) -> (0, 173.7399)
  line L3 (0, 173.7399) -> (-6, 173.7399)
  line L4 (608, 158.7399) -> (608, 173.7399)
  line L5 (608, 173.7399) -> (602, 173.7399)
  line L6 (602, 173.7399) -> (602, 158.7399)
  line L7 (602, 158.7399) -> (608, 158.7399)
  line L8 (0, -35.13) -> (0, -27.13)
  line L9 (0, -27.13) -> (-12, -27.13)
  line L10 (-12, -27.13) -> (-12, -35.13)
  line L11 (-12, -35.13) -> (0, -35.13)
  line L12 (0, -56.13) -> (0, -48.13)
  line L13 (0, -48.13) -> (-12, -48.13)
  line L14 (-12, -48.13) -> (-12, -56.13)
  line L15 (-12, -56.13) -> (0, -56.13)
  line L16 (602, -27.13) -> (602, -35.13)
  line L17 (602, -35.13) -> (614, -35.13)
  line L18 (614, -35.13) -> (614, -27.13)
  line L19 (614, -27.13) -> (602, -27.13)
  line L20 (602, -48.13) -> (602, -56.13)
  line L21 (602, -56.13) -> (614, -56.13)
  line L22 (614, -56.13) -> (614, -48.13)
  line L23 (614, -48.13) -> (602, -48.13)
  line L24 (-6, 158.7399) -> (-6, 150.7399)
  line L25 (-6, 150.7399) -> (0, 150.7399)
  line L26 (0, 150.7399) -> (0, 158.7399)
  line L27 (0, 158.7399) -> (-6, 158.7399)
  line L28 (608, 150.7399) -> (608, 158.7399)
  line L29 (608, 158.7399) -> (602, 158.7399)
  line L30 (602, 158.7399) -> (602, 150.7399)
  line L31 (602, 150.7399) -> (608, 150.7399)
  line L32 (-6, 164.7399) -> (0, 164.7399)
  line L33 (0, 164.7399) -> (0, 158.7399)
  line L34 (0, 158.7399) -> (-6, 158.7399)
  line L35 (-6, 158.7399) -> (-6, 164.7399)
  line L36 (602, 158.7399) -> (608, 158.7399)
  line L37 (608, 158.7399) -> (608, 164.7399)
  line L38 (608, 164.7399) -> (602, 164.7399)
  line L39 (602, 164.7399) -> (602, 158.7399)
  line L40 (0, 164.7399) -> (602, 164.7399)
  line L41 (602, 164.7399) -> (602, -47.63)
  line L42 (602, -47.63) -> (0, -47.63)
  line L43 (0, -47.63) -> (0, 164.7399)
  line L44 (614, -35.13) -> (614, -48.13)
  line L45 (-12, -35.13) -> (-12, -48.13)
  line L46 (602, -35.13) -> (614, -35.13)
  line L47 (614, -35.13) -> (614, -48.13)
  line L48 (614, -48.13) -> (602, -48.13)
  line L49 (602, -48.13) -> (602, -35.13)
  line L50 (0, -35.13) -> (-12, -35.13)
  line L51 (-12, -35.13) -> (-12, -48.13)
  line L52 (-12, -48.13) -> (0, -48.13)
  line L53 (0, -48.13) -> (0, -35.13)
  line L54 (-12, -36.0852) -> (0, -36.0852)
  line L55 (0, -36.0852) -> (0, -47.63)
  line L56 (0, -47.63) -> (-12, -47.63)
  line L57 (-12, -47.63) -> (-12, -36.0852)
  line L58 (602, -47.63) -> (614, -47.63)
  line L59 (614, -47.63) -> (614, -35.63)
  line L60 (614, -35.63) -> (602, -35.63)
  line L61 (602, -35.63) -> (602, -47.63)
  spline S0 degree 5 poles (69.933, 164.7399) (70.4919, 159.1631) (71.7193, 148.2006) (73.8887, 132.3304) (77.6335, 112.4801) (84.808, 90.7425) (95.7159, 73.0853) (111.3868, 60.2852) (132.0599, 52.3455) (156.9705, 48.3011) (184.937, 46.7974) (208.7318, 46.4893) (226.9175, 46.2548) (239.1314, 46.0302) (245.261, 45.9008) knots 0 0 0 0 0 0 0.1 0.2 0.3 0.4 0.5 0.6 0.7 0.8 0.9 1 1 1 1 1 1
  line L62 (301, 164.7399) -> (301, -47.63)
  line L63 (245.261, 45.9008) -> (301, 45.9008)
  spline S1 degree 5 poles (532.067, 164.7399) (531.5081, 159.1631) (530.2807, 148.2006) (528.1113, 132.3304) (524.3665, 112.4801) (517.192, 90.7425) (506.2841, 73.0853) (490.6132, 60.2852) (469.9401, 52.3455) (445.0295, 48.3011) (417.063, 46.7974) (393.2682, 46.4893) (375.0825, 46.2548) (362.8686, 46.0302) (356.739, 45.9008) knots 0 0 0 0 0 0 0.1 0.2 0.3 0.4 0.5 0.6 0.7 0.8 0.9 1 1 1 1 1 1
  line L64 (67.0686, 193.3182) -> (72.7974, 136.1616)
  line L65 (217.6221, 46.4842) -> (272.8999, 45.3174)
  line L66 (534.9314, 193.3182) -> (529.2026, 136.1616)
  line L67 (384.378, 46.4842) -> (329.1001, 45.3174)
  line L68 (356.739, 45.9008) -> (301, 45.9008)
  line L69 (-12, -56.13) -> (0, -56.13)
  line L70 (0, -56.13) -> (0, -44.13)
  line L71 (0, -44.13) -> (-12, -44.13)
  line L72 (-12, -44.13) -> (-12, -56.13)
  line L73 (602, -44.13) -> (614, -44.13)
  line L74 (0, -56.13) -> (602, -56.13)
  line L75 (614, -56.13) -> (602, -56.13)
  line L76 (602, -56.13) -> (602, -44.13)
  line L77 (602, -44.13) -> (614, -44.13)
  line L78 (614, -44.13) -> (614, -56.13)
  line L79 (0, -56.13) -> (-12, -56.13)
  line L80 (-12, -56.13) -> (-12, -44.13)
  line L81 (-12, -44.13) -> (0, -44.13)
  line L82 (0, -44.13) -> (0, -56.13)
  point P0 (106.6702, 65.3557)
  point P1 (495.3298, 65.3557)
  dimension "d106" = 14
  dimension "d107" = 0.5
  dimension "d112" = 12
  dimension "d196" = 12
  constraint horizontal L32
  constraint vertical L33
  constraint horizontal L34
  constraint vertical L35
  constraint coincident L1.end L2.start
  constraint coincident L0 L32.start
  constraint horizontal L36
  constraint vertical L37
  constraint horizontal L38
  constraint vertical L39
  constraint coincident L4 L37.end
  constraint coincident L6.end L7.start
  constraint collinear L32 L38
  constraint horizontal L40
  constraint vertical L41
  constraint horizontal L42
  constraint vertical L43
  constraint coincident L17.end L18.start
  constraint coincident L22.end L23.start
  constraint coincident L10.end L11.start
  constraint coincident L13.end L14.start
  constraint horizontal L46
  constraint vertical L47
  constraint horizontal L48
  constraint vertical L49
  constraint coincident L16.end L17.start
  constraint horizontal L50
  constraint vertical L51
  constraint horizontal L52
  constraint vertical L53
  constraint coincident L8.start L11.end
  constraint horizontal L54
  constraint vertical L55
  constraint horizontal L56
  constraint vertical L57
  constraint coincident L51 L54.start
  constraint horizontal L58
  constraint vertical L59
  constraint horizontal L60
  constraint vertical L61
  constraint coincident L40 S0.start
  constraint midpoint L40 L62.start
  constraint midpoint L42 L62.end
  constraint horizontal L63
  constraint midpoint S0.start L64
  constraint midpoint S0.end L65
  constraint symmetric S0.start L62 S1.start
  constraint symmetric P0 L62 P1
  constraint symmetric S0.end L62 S1.end
  constraint symmetric L62 L63.end L68.end
  constraint symmetric L62 L64.start L66.start
  constraint symmetric L62 L64.end L66.end
  constraint symmetric L62 L65.start L67.start
  constraint symmetric L62 L65.end L67.end
  constraint coincident L62 L63.end
  constraint horizontal L69
  constraint vertical L70
  constraint horizontal L71
  constraint vertical L72
  constraint coincident L53 L70.end
  constraint coincident L14.end L15.start
  constraint coincident L49 L73.start
  constraint coincident L44 L73.end
  constraint perpendicular L44 L73
  constraint collinear L71 L73
  constraint coincident L12.start L15.end
  constraint coincident L20.end L21.start
  constraint horizontal L75
  constraint vertical L76
  constraint horizontal L77
  constraint vertical L78
  constraint coincident L21.end L22.start
  constraint horizontal L79
  constraint vertical L80
  constraint horizontal L81
  constraint vertical L82
  measures "d106" distance of L31 L38
  measures "d107" distance of L20.start L41.end
  measures "d112" distance of L41.end L60.end
  measures "d196" distance of L69 L71
extrude "Extrusion14" add sketch "Esquisse6" along normal blind 12 separate body contours L0 L1 L2 L27 L32 L33 L34 L35 L43 | L1 L24 L25 L26 L27 L34 L43 | L2 L8 L26 L33 L40 L42 L43 L53 L55 S0 L62 L63 L70 L82 | L6 L16 L30 L39 L40 L41 L42 L49 L61 L62 S1 L68 L76 | L4 L6 L7 L29 L36 L37 L38 L39 L41 | L12 L20 L42 L49 L53 L70 L74 L76 L82 | L7 L28 L29 L30 L31 L36 L41 | L23 L44 L47 L48 L49 L58 L76 L78 | L41 L44 L47 L49 L58 L59 L61 L73 L76 L77 L78 | L43 L45 L51 L53 L55 L56 L57 L70 L71 L72 L80 L81 L82 | L13 L45 L51 L52 L53 L56 L70 L72 L80 L82 | L20 L21 L22 L23 L48 L75 L76 L78 | L12 L13 L14 L15 L52 L69 L70 L72 L79 L80 L82 makes body 6
combine "Combiner3" operation cut target body 6 tool bodies 1 keep tools
combine "Combiner4" operation cut target body 6 tool bodies 2 keep tools
sketch "Esquisse7" plane through (-602, 0, 0) normal (1, 0, 0) x (0, 0, 1)
  line L0 (-59, 12) -> (-59, 0)
  line L1 (-59, 0) -> (-150, 0)
  line L2 (-150, 0) -> (-150, 12)
  line L3 (-150, 12) -> (-59, 12)
  line L4 (-180, -273.7143) -> (-192, -273.7143)
  line L5 (-192, -273.7143) -> (-192, -130.8571)
  line L6 (-192, -130.8571) -> (-180, -130.8571)
  line L7 (-180, -130.8571) -> (-180, -273.7143)
  line L8 (-180, -416.5714) -> (-180, -559.4286)
  line L9 (-180, -559.4286) -> (-192, -559.4286)
  line L10 (-192, -559.4286) -> (-192, -416.5714)
  line L11 (-192, -416.5714) -> (-180, -416.5714)
  line L12 (0, -845.1428) -> (0, -702.2857)
  line L13 (0, -702.2857) -> (12, -702.2857)
  line L14 (12, -702.2857) -> (12, -845.1428)
  line L15 (12, -845.1428) -> (0, -845.1428)
  line L16 (-241, 12) -> (-241, 0)
  line L17 (-241, 0) -> (-332, 0)
  line L18 (-332, 0) -> (-332, 12)
  line L19 (-332, 12) -> (-241, 12)
  line L20 (0, -273.7143) -> (0, -130.8571)
  line L21 (0, -130.8571) -> (12, -130.8571)
  line L22 (12, -130.8571) -> (12, -273.7143)
  line L23 (12, -273.7143) -> (0, -273.7143)
  line L24 (-180, -702.2857) -> (-180, -845.1428)
  line L25 (-180, -845.1428) -> (-192, -845.1428)
  line L26 (-192, -845.1428) -> (-192, -702.2857)
  line L27 (-192, -702.2857) -> (-180, -702.2857)
  line L28 (0, -559.4286) -> (0, -416.5714)
  line L29 (0, -416.5714) -> (12, -416.5714)
  line L30 (12, -416.5714) -> (12, -559.4286)
  line L31 (12, -559.4286) -> (0, -559.4286)
  line L32 (-423, 12) -> (-423, 0)
  line L33 (-423, 0) -> (-514, 0)
  line L34 (-514, 0) -> (-514, 12)
  line L35 (-514, 12) -> (-423, 12)
  line L36 (-593, 35.13) -> (-593, 27.13)
  line L37 (-593, 27.13) -> (-605, 27.13)
  line L38 (-605, 27.13) -> (-605, 35.13)
  arc A0 (-605, 48.13) -> (-605, 35.13) centre (-599, 41.63) ccw
  line L39 (-605, 48.13) -> (-605, 56.13)
  line L40 (-605, 56.13) -> (-593, 56.13)
  line L41 (-593, 56.13) -> (-593, 48.13)
  arc A1 (-593, 35.13) -> (-593, 48.13) centre (-599, 41.63) ccw
  circle A2 centre (6, -115.8571) radius 2
  circle A3 centre (-161.8713, 6) radius 2
  circle A4 centre (6, -288.7143) radius 2
  circle A5 centre (6, -401.5714) radius 2
  circle A6 centre (-229, 6) radius 2
  circle A7 centre (-343.8713, 6) radius 2
  circle A8 centre (6, -574.4286) radius 2
  circle A9 centre (6, -687.2857) radius 2
  circle A10 centre (6, -860.1428) radius 2
  circle A11 centre (-525.8713, 6) radius 2
  circle A12 centre (-581, 6) radius 2
  circle A13 centre (-186, -687.2857) radius 2
  circle A14 centre (-411, 6) radius 2
  circle A15 centre (6, -15) radius 2
  circle A16 centre (6, -973) radius 2
  circle A17 centre (-186, -288.7143) radius 2
  circle A18 centre (-186, -860.1428) radius 2
  circle A19 centre (-186, -973) radius 2
  circle A20 centre (-186, -401.5714) radius 2
  circle A21 centre (-186, -574.4286) radius 2
  circle A22 centre (-186, -15) radius 2
  circle A23 centre (-186, -115.8571) radius 2
  circle A24 centre (20.1287, 6) radius 2
  circle A25 centre (-47, 6) radius 2
  arc A26 (-585.3674, 68.3537) -> (-626.1765, 28.9242) centre (-599, 41.63) ccw
  line L42 (-626.1765, 28.9242) -> (-605, -16.37)
  line L43 (-605, -16.37) -> (-605, -158.7399)
  line L44 (-605, -158.7399) -> (-599, -158.7399)
  line L45 (-599, -158.7399) -> (-599, -150.7399)
  line L46 (-599, -150.7399) -> (-593, -150.7399)
  line L47 (-593, -150.7399) -> (-593, -158.7399)
  line L48 (-593, -158.7399) -> (-593, -173.7399)
  line L49 (-593, -173.7399) -> (-605, -173.7399)
  arc A27 (-605, -173.7399) -> (-569.8721, -317.6877) centre (-292.5, -173.7399) ccw
  line L50 (-569.8721, -317.6877) -> (-227.5983, -977.2127)
  arc A28 (-227.5983, -977.2127) -> (-209.8465, -988) centre (-209.8465, -968) ccw
  line L51 (-209.8465, -988) -> (32.1287, -988)
  line L52 (32.1287, -988) -> (32.1287, 12)
  line L53 (32.1287, 12) -> (32, 12)
  line L54 (32, 12) -> (32, 32)
  line L55 (32, 32) -> (-514.1044, 32)
  line L56 (-514.1044, 32) -> (-585.3674, 68.3537)
  point P0 (-61.3335, 9.6665)
  point P1 (-61.3335, 2.3335)
  point P2 (-147.6665, 2.3335)
  point P3 (-147.6665, 9.6665)
  point P4 (-182.3335, -271.3808)
  point P5 (-189.6665, -271.3808)
  point P6 (-189.6665, -133.1906)
  point P7 (-182.3335, -133.1906)
  point P8 (-182.3335, -418.9049)
  point P9 (-182.3335, -557.0951)
  point P10 (-189.6665, -557.0951)
  point P11 (-189.6665, -418.9049)
  point P12 (2.3335, -842.8094)
  point P13 (2.3335, -704.6192)
  point P14 (9.6665, -704.6192)
  point P15 (9.6665, -842.8094)
  point P16 (-243.3335, 9.6665)
  point P17 (-243.3335, 2.3335)
  point P18 (-329.6665, 2.3335)
  point P19 (-329.6665, 9.6665)
  point P20 (2.3335, -271.3808)
  point P21 (2.3335, -133.1906)
  point P22 (9.6665, -133.1906)
  point P23 (9.6665, -271.3808)
  point P24 (-182.3335, -704.6192)
  point P25 (-182.3335, -842.8094)
  point P26 (-189.6665, -842.8094)
  point P27 (-189.6665, -704.6192)
  point P28 (2.3335, -557.0951)
  point P29 (2.3335, -418.9049)
  point P30 (9.6665, -418.9049)
  point P31 (9.6665, -557.0951)
  point P32 (-425.3335, 9.6665)
  point P33 (-425.3335, 2.3335)
  point P34 (-511.6665, 2.3335)
  point P35 (-511.6665, 9.6665)
  point P36 (-595.3335, 29.4635)
  point P37 (-602.6665, 29.4635)
  point P38 (-595.3335, 53.7966)
  point P39 (-602.6665, 53.7966)
  point P40 (-608.2214, -17.0858)
  point P41 (-513.3333, 35.2086)
  point P42 (-595.3335, -153.0734)
  point P43 (-596.6665, -153.0734)
  point P44 (34.3335, 14.3335)
  point P45 (-595.3335, -171.4065)
fillet "Congé3" radius 40 2 edges at (-69.933, 164.7399, -599) (-532.067, 164.7399, -599) on bodies 6
fillet "Congé2" radius 20 2 edges at (6, -32, 32) (-608, -32, 32) on bodies 1 2
fillet "Congé2" radius 20 2 edges at (6, 988, 32.1287) (-608, 988, 32.1287) on bodies 1 2